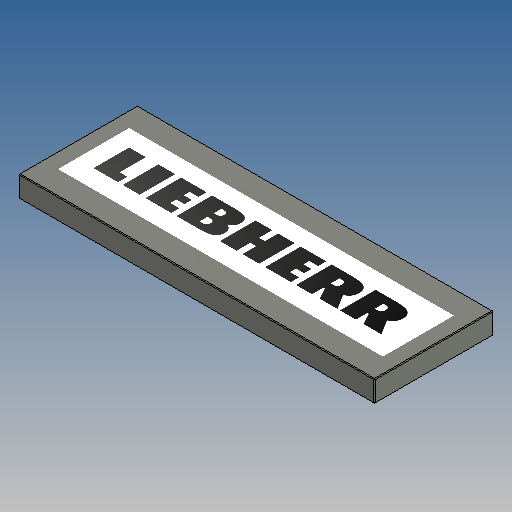
# Autodesk Inventor part: 69729-DkBluishGray
Saved by Autodesk Inventor 2025 (Build 290162010, 162A)
## iProperties
Created: 2014-06-03
Part Number: 69729-DkBluishGray
Material: ABS Plastic
Document SubType Name: Modeling
Designer: h.muther
Density: 1.06 g/cm^3
Appearance: DkBluishGray
Mass: 1.17272 g
Surface Area: 16.2903 cm^2
Volume: 1.10634 cm^3
Author: h.muther
Autodesk Inventor part; units mm, degrees
ref_plane "YZ Plane" through (0, 0, 0) normal (1, 0, 0) x (0, 1, 0)
ref_plane "XZ Plane" through (0, 0, 0) normal (0, 1, 0) x (-1, 0, 0)
ref_plane "XY Plane" through (0, 0, 0) normal (0, 0, 1) x (1, 0, 0)
sketch "Sketch2" plane through (0, 0, 0) normal (0, 1, 0) x (-1, 0, 0)
  line L0 (-24, 8) -> (24, 8)
  line L1 (24, 8) -> (24, -8)
  line L2 (24, -8) -> (-24, -8)
  line L3 (-24, -8) -> (-24, 8)
  point P0 (0, 0)
  point P1 (0, 8)
  point P2 (-24, 0)
  dimension "d0" = 48
  dimension "d1" = 16
  constraints: 8 end point, 2 midpoint, 2 parallel, 1 horizontal, 1 horizontal alignment, 1 perpendicular, 1 vertical alignment
  measures "d0" distance of L1.end L2.end
  measures "d1" distance of L2.end L0.start
extrude "Extrusion1" add sketch "Sketch2" along normal blind 3.2
sketch "Sketch3" plane through (0, 0, 0) normal (0, -1, 0) x (1, 0, 0)
  line L0 (-24, 8) -> (-24, -8) projected
  line L1 (-22.4, 6.4) -> (22.4, 6.4)
  line L2 (22.4, 6.4) -> (22.4, -6.4)
  line L3 (22.4, -6.4) -> (-22.4, -6.4)
  line L4 (-22.4, -6.4) -> (-22.4, 6.4)
  circle A0 centre (-16, 0) radius 3.2569
  circle A1 centre (-16, 0) radius 2.4
  line L5 (-24, -8) -> (24, -8) projected
  circle A2 centre (0, 0) radius 1.6
  line L6 (24, -8) -> (24, 8) projected
  line L7 (-12, 0) -> (-4, 0) construction
  line L8 (-4, 0) -> (4, 0) construction
  line L9 (4, 0) -> (12, 0) construction
  circle A3 centre (-20, 4) radius 2.4 construction
  circle A4 centre (-20, -4) radius 2.4 construction
  circle A5 centre (20, -4) radius 2.4 construction
  circle A6 centre (20, 4) radius 2.4 construction
  line L10 (24, 8) -> (-24, 8) projected
  line L11 (-23.6, 7.6) -> (23.6, 7.6)
  line L12 (23.6, 7.6) -> (23.6, -7.6)
  line L13 (23.6, -7.6) -> (-23.6, -7.6)
  line L14 (-23.6, -7.6) -> (-23.6, 7.6)
  point P0 (-22.4, 0)
  point P1 (0, 6.4)
  point P2 (0, 0)
  point P3 (0, 7.6)
  point P4 (-23.6, 0)
  dimension "d61" = 4.8
  dimension "d75" = 8
  dimension "d76" = 8
  dimension "d86" = 3.2
  dimension "d92" = 8
  dimension "d98" = 40
  dimension "d99" = 8
  dimension "d102" = 0.4
  dimension "d103" = 0.4
  constraints: 22 end point, 9 tangent, 7 centre point, 6 equal length, 5 midpoint, 4 equal radius, 3 coincident, 3 perpendicular, 2 collinear, 2 horizontal, 2 horizontal alignment, 2 vertical alignment
  measures "d61" diameter of A1
  measures "d75" distance from line of A0.centre L0
  measures "d76" distance from line of A0.centre L5
  measures "d86" diameter of A2
  measures "d92" distance of L7.end L8.end
  measures "d98" distance of A6.centre A3.centre
  measures "d99" distance of A4.centre A3.centre
  measures "d102" distance between parallel lines of L11 L10
  measures "d103" distance between parallel lines of L0 L14
extrude "Extrusion2" cut sketch "Sketch3" against normal blind 1.6 contours L1 L2 L3 L4 | A0 | A1 | A2
extrude "Extrusion7" cut sketch "Sketch3" against normal blind 0.4 contours L10 L6 L5 L0
extrude "Extrusion6" add sketch "Sketch3" against normal up to next contours A0
pattern_linear "Rectangular Pattern3" count 5 spacing 8 along (1, 0, 0) of "Extrusion6"
fillet "Fillet1" radius 0.1 8 edges at (-24, 1.8, 8) (0, 3.2, 8) (-24, 3.2, 0) (0, 3.2, -8) (24, 3.2, 0) (24, 1.8, 8) (24, 1.8, -8) (-24, 1.8, -8)
sketch "Skizze10" plane through (0, 3.2, 0) normal (0, 1, 0) x (1, 0, 0)
  line L0 (-21.913, 4.8) -> (21.913, 4.8) construction
  line L1 (21.913, 4.8) -> (21.913, -4.8) construction
  line L2 (21.913, -4.8) -> (-21.913, -4.8) construction
  line L3 (-21.913, -4.8) -> (-21.913, 4.8) construction
  line L4 (23.9, 8) -> (-23.9, 8) projected
  line L5 (-23.9, -8) -> (23.9, -8) projected
  point P0 (0, 0)
  point P1 (0, 4.8)
  point P2 (0, 8)
  dimension "d107" = 3.2
  dimension "d110" = 3.2
  constraints: 2 midpoint, 1 vertical alignment, 2 other
  measures "d107" distance between parallel lines of L4 L0
  measures "d110" distance between parallel lines of L2 L5
decal "Aufkleber1"
equation "\"d4\" = 0.333333 * lh"
equation "\"d61\" = kd"
equation "\"d75\" = lu"
equation "\"d76\" = d75"
equation "\"d86\" = pd"
equation "\"d92\" = lu"
equation "\"d98\" = 5 * lu"
equation "\"d99\" = d75"
equation "\"d102\" = gw"
equation "\"d103\" = gw"
equation "\"d11\" = 0.333333 * lh - topthk"
equation "\"d104\" = gh"
equation "\"d91\" = lu"
equation "\"d110\" = d107"
equation "\"lh\" = 9.6"
equation "\"kd\" = 4.8"
equation "\"lu\" = 8"
equation "\"pd\" = 3.2"
equation "\"gw\" = 0.4"
equation "\"topthk\" = 1.6"
equation "\"gh\" = 0.4"
body "Solid1"
